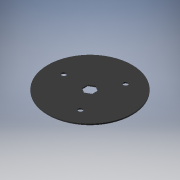
# Autodesk Inventor part: spoolEnd
Saved by Autodesk Inventor 2017 (Build 210142000, 142)
## iProperties
Created: 2017-03-09
Part Number: spoolEnd
Material: Generic
Document SubType Name: Modeling
Designer: kingb
Density: 1 g/cm^3
Appearance: Default
Author: kingb
Autodesk Inventor part; units mm, degrees
ref_plane "YZ Plane" through (0, 0, 0) normal (1, 0, 0) x (0, 1, 0)
ref_plane "XZ Plane" through (0, 0, 0) normal (0, 1, 0) x (-1, 0, 0)
ref_plane "XY Plane" through (0, 0, 0) normal (0, 0, 1) x (1, 0, 0)
sketch "Sketch1" plane through (0, 0, 0) normal (0, 1, 0) x (-1, 0, 0)
  line L0 (6.35, -3.6662) -> (0, -7.3323)
  line L1 (0, -7.3323) -> (-6.35, -3.6662)
  line L2 (-6.35, -3.6662) -> (-6.35, 3.6662)
  line L3 (-6.35, 3.6662) -> (0, 7.3323)
  line L4 (0, 7.3323) -> (6.35, 3.6662)
  line L5 (6.35, 3.6662) -> (6.35, -3.6662)
  circle A0 centre (0, 0) radius 38.1
  line L6 (31.5732, -7.3323) -> (25.2232, -3.6662)
  line L7 (25.2232, -3.6662) -> (25.2232, 3.6662)
  line L8 (25.2232, 3.6662) -> (31.5732, 7.3323)
  line L9 (31.5732, 7.3323) -> (37.9232, 3.6662)
  line L10 (37.9232, 3.6662) -> (37.9232, -3.6662)
  line L11 (37.9232, -3.6662) -> (31.5732, -7.3323)
  line L12 (-15.7866, -20.0108) -> (-9.4366, -23.677)
  line L13 (-9.4366, -23.677) -> (-9.4366, -31.0094)
  line L14 (-9.4366, -31.0094) -> (-15.7866, -34.6755)
  line L15 (-15.7866, -34.6755) -> (-22.1366, -31.0094)
  line L16 (-22.1366, -31.0094) -> (-22.1366, -23.677)
  line L17 (-22.1366, -23.677) -> (-15.7866, -20.0108)
  line L18 (-15.7866, 20.0108) -> (-22.1366, 23.677)
  line L19 (-22.1366, 23.677) -> (-22.1366, 31.0094)
  line L20 (-22.1366, 31.0094) -> (-15.7866, 34.6755)
  line L21 (-15.7866, 34.6755) -> (-9.4366, 31.0094)
  line L22 (-9.4366, 31.0094) -> (-9.4366, 23.677)
  line L23 (-9.4366, 23.677) -> (-15.7866, 20.0108)
  circle A1 centre (0, 0) radius 50.8
  circle A2 centre (31.5732, 0) radius 2.9337
  circle A3 centre (-15.7866, -27.3432) radius 2.9337
  circle A4 centre (-15.7866, 27.3432) radius 2.9337
  dimension "d0" = 6.35
  dimension "d1" = 76.2
  dimension "d2" = 120
  dimension "d3" = 120
  dimension "d4" = 12.7
  dimension "d5" = 5.8674
  constraints: 48 end point, 6 point on circle, 5 centre point, 5 coincident, 3 equal length, 2 equal radius, 1 parallel, 1 vertical alignment, 52 other
  measures "d0" distance from line of point (0, 0) L5
  measures "d1" diameter of A0
  measures "d4" radial gap between concentric circles of A0 A1
  measures "d5" diameter of A2
extrude "Extrusion1" add sketch "Sketch1" along normal blind 1.5875 contours A0 L10 | L9 L8 L7 L6 L11 A0 L14 L13 L12 L17 L16 L19 L18 L23 L22 L21 | L10 L11 L6 L7 L8 L9 | L20 A0 | L21 L22 L23 L18 L19 L20 | L15 L16 L17 L12 L13 L14 | A0 L15 | A1
body "Solid1"
